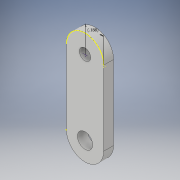
# Autodesk Inventor part: Part5
Saved by Autodesk Inventor 2019 (Build 230136000, 136)
## iProperties
Created: 2019-05-23
Part Number: Part5
Material: Generic
Document SubType Name: Modeling
Designer: bgereke
Density: 1 g/cm^3
Appearance: Default
Author: bgereke
Autodesk Inventor part; units mm, degrees
ref_plane "YZ Plane" through (0, 0, 0) normal (1, 0, 0) x (0, 1, 0)
ref_plane "XZ Plane" through (0, 0, 0) normal (0, 1, 0) x (-1, 0, 0)
ref_plane "XY Plane" through (0, 0, 0) normal (0, 0, 1) x (1, 0, 0)
sketch "Sketch1" plane through (0, 0, 0) normal (0, 0, 1) x (1, 0, 0)
  line L0 (9.525, 0) -> (9.525, 19.05)
  line L1 (0, 19.05) -> (0, 0)
  arc A0 (9.525, 19.05) -> (0, 19.05) centre (4.7625, 19.05) ccw
  arc A1 (0, 0) -> (9.525, 0) centre (4.7625, 0) ccw
  dimension "d0" = 9.525
  dimension "d1" = 19.05
  constraints: 4 end point, 4 point on circle, 2 centre point, 1 parallel
  measures "d0" distance of L1.start L0.end
  measures "d1" distance of L0.end L0.start
extrude "Extrusion1" add sketch "Sketch1" along normal blind 2.54
sketch "Sketch2" plane through (0, 0, 2.54) normal (0, 0, 1) x (1, 0, 0)
  arc A0 (9.525, 19.05) -> (0, 19.05) centre (4.7625, 19.05) ccw projected
  point P0 (0, 0)
  dimension "d18" = 4.7625
  constraints: 1 coincident
  measures "d18" distance of A0.centre A0.start
hole "Hole1" at (4.7625, 19.05, 2.54) direction (0, 0, -1) diameter 2.9 end through all
sketch "Sketch3" plane through (0, 0, 2.54) normal (0, 0, 1) x (1, 0, 0)
  circle A0 centre (4.7625, 19.05) radius 1.45 projected
  point P0 (0, 0)
  point P1 (4.7752, 0)
  dimension "d19" = 4.7752
  dimension "d20" = 19.05
  dimension "d21" = 2.9
  measures "d19" distance of point (0, 0) point (4.775, 0)
  measures "d20" distance of point (4.775, 0) A0.centre
  measures "d21" diameter of A0
hole "Hole2" at (4.7752, 0, 2.54) direction (0, 0, -1) diameter 3.9 end through all
body "Solid1"
